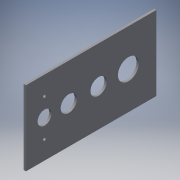
# Autodesk Inventor part: ARm Gearbox Plate
Saved by Autodesk Inventor 2018 (Build 220112000, 112)
## iProperties
Created: 2019-01-19
Part Number: ARm Gearbox Plate
Material: Generic
Document SubType Name: Modeling
Designer: Gabriel
Density: 1 g/cm^3
Appearance: Default
Author: Gabriel
Autodesk Inventor part; units mm, degrees
ref_plane "YZ Plane" through (0, 0, 0) normal (1, 0, 0) x (0, 1, 0)
ref_plane "XZ Plane" through (0, 0, 0) normal (0, 1, 0) x (-1, 0, 0)
ref_plane "XY Plane" through (0, 0, 0) normal (0, 0, 1) x (1, 0, 0)
sketch "Sketch1" plane through (0, 0, 0) normal (1, 0, 0) x (0, 1, 0)
  line L0 (86.7421, 202.4896) -> (-14.8579, 202.4896)
  line L1 (-14.8579, 202.4896) -> (-14.8579, 24.6896)
  line L2 (-14.8579, 24.6896) -> (86.7421, 24.6896)
  line L3 (86.7421, 24.6896) -> (86.7421, 202.4896)
  line L4 (86.7421, 202.4896) -> (86.7421, 227.8896) construction
  point P0 (0, 0)
  dimension "d0" = 101.6
  dimension "d1" = 177.8
  dimension "d23" = 25.4
  constraints: 10 end point, 2 parallel, 1 horizontal, 1 perpendicular, 1 vertical
  measures "d0" distance of L2.end L1.end
  measures "d1" distance of L1.end L0.end
  measures "d23" distance of L0.start L4.end
extrude "Extrusion1" add sketch "Sketch1" along normal blind 3.175
sketch "Sketch2" plane through (3.175, 0, 0) normal (1, 0, 0) x (0, 0, -1)
  line L0 (-202.4896, 86.7421) -> (-202.4896, -14.8579) construction
  line L1 (-202.4896, 35.9421) -> (-177.0896, 35.9421) construction
  line L2 (-177.0896, 35.9421) -> (-144.0696, 35.9421) construction
  circle A0 centre (-144.0696, 35.9421) radius 11.1125
  line L3 (-144.0696, 35.9421) -> (-103.4296, 35.9421) construction
  line L4 (-103.4296, 35.9421) -> (-62.7896, 35.9421) construction
  circle A1 centre (-103.4296, 35.9421) radius 11.1125
  circle A2 centre (-62.7896, 35.9421) radius 14.2875
  circle A3 centre (-177.0896, 35.9421) radius 9.525
  point P0 (0, 0)
  dimension "d4" = 25.4
  dimension "d5" = 33.02
  dimension "d7" = 22.225
  dimension "d8" = 40.64
  dimension "d9" = 40.64
  dimension "d10" = 22.225
  dimension "d11" = 28.575
  dimension "d14" = 19.05
  constraints: 8 end point, 4 centre point, 4 coincident, 3 horizontal, 1 midpoint, 1 point on line
  measures "d4" distance of L1.start L1.end
  measures "d5" distance of L1.end L2.end
  measures "d7" diameter of A0
  measures "d8" distance of L3.start L3.end
  measures "d9" distance of L3.end L4.end
  measures "d10" diameter of A1
  measures "d11" diameter of A2
  measures "d14" diameter of A3
extrude "Extrusion2" cut sketch "Sketch2" against normal blind 12.7
sketch "Sketch3" plane through (0, 0, 0) normal (-1, 0, 0) x (0, 0, 1)
  circle A0 centre (177.0896, 35.9421) radius 9.525 projected
  circle A1 centre (177.0836, 61.3421) radius 2.0193
  circle A2 centre (177.0836, 10.5421) radius 2.0193
  line L0 (177.0836, 61.3421) -> (177.0836, 10.5421) construction
  point P0 (0, 0)
  dimension "d17" = 4.0386
  dimension "d18" = 4.0386
  constraints: 2 centre point, 2 end point, 1 vertical
  measures "d17" diameter of A1
  measures "d18" diameter of A2
extrude "Extrusion3" cut sketch "Sketch3" against normal blind 25.4 contours A1 | A2
sketch "Sketch4" plane through (3.175, 0, 0) normal (1, 0, 0) x (0, 0, -1)
  line L0 (-24.6896, 86.7421) -> (-202.4896, 86.7421) construction
  line L1 (-202.4896, 86.7421) -> (-189.7896, 86.7421) construction
  line L2 (-189.7896, 86.7421) -> (-189.7896, 74.0421) construction
  line L3 (-189.7896, 74.0421) -> (-202.4896, 74.0421) construction
  line L4 (-202.4896, 74.0421) -> (-202.4896, 86.7421) construction
  line L5 (-202.4896, 86.7421) -> (-202.4896, -14.8579) construction
  line L6 (-202.4896, -14.8579) -> (-189.7896, -14.8579) construction
  line L7 (-189.7896, -14.8579) -> (-189.7896, -2.1579) construction
  line L8 (-189.7896, -2.1579) -> (-202.4896, -2.1579) construction
  line L9 (-202.4896, -2.1579) -> (-202.4896, -14.8579) construction
  line L10 (-202.4896, -14.8579) -> (-24.6896, -14.8579) construction
  line L11 (-24.6896, -14.8579) -> (-37.3896, -14.8579) construction
  line L12 (-37.3896, -14.8579) -> (-37.3896, -2.1579) construction
  line L13 (-37.3896, -2.1579) -> (-24.6896, -2.1579) construction
  line L14 (-24.6896, -2.1579) -> (-24.6896, -14.8579) construction
  line L15 (-24.6896, 86.7421) -> (-37.3896, 86.7421) construction
  line L16 (-37.3896, 86.7421) -> (-37.3896, 74.0421) construction
  line L17 (-37.3896, 74.0421) -> (-24.6896, 74.0421) construction
  line L18 (-24.6896, 74.0421) -> (-24.6896, 86.7421) construction
  circle A0 centre (-189.7896, 74.0421) radius 2.54
  circle A1 centre (-37.3896, 74.0421) radius 2.54
  circle A2 centre (-37.3896, -2.1579) radius 2.54
  circle A3 centre (-189.7896, -2.1579) radius 2.54
  point P0 (0, 0)
  dimension "d24" = 12.7
  dimension "d25" = 12.7
  dimension "d26" = 12.7
  dimension "d27" = 12.7
  dimension "d28" = 12.7
  dimension "d29" = 12.7
  dimension "d30" = 12.7
  dimension "d31" = 12.7
  dimension "d32" = 5.08
  dimension "d33" = 5.08
  dimension "d34" = 5.08
  dimension "d35" = 5.08
  constraints: 32 end point, 8 parallel, 4 centre point, 4 coincident, 4 horizontal, 4 perpendicular, 2 point on line
  measures "d24" distance of L2.end L3.end
  measures "d25" distance of L1.end L2.end
  measures "d26" distance of L8.end L7.end
  measures "d27" distance of L7.end L6.end
  measures "d28" distance of L12.end L13.end
  measures "d29" distance of L11.end L12.end
  measures "d30" distance of L17.end L16.end
  measures "d31" distance of L16.end L15.end
  measures "d32" diameter of A0
  measures "d33" diameter of A1
  measures "d34" diameter of A2
  measures "d35" diameter of A3
extrude "Extrusion4" cut sketch "Sketch4" against normal blind 25.4
body "Solid1"
